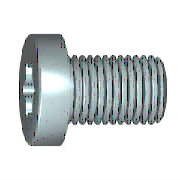
# Autodesk Inventor part: NF E 25-111 - M8x30 classe proprietà 4.8
Saved by Autodesk Inventor 2022 (Build 260153000, 153)
## iProperties
Created: 2021-02-02
Part Number: NF E 25-111 - M8x30 classe proprietà 4.8
Material: Acciaio, Dolce
Description: Testa svasata con impronta a sei lobi - Grado prodotto A - Simbolo CZX
Document SubType Name: Modeling
Standard: NF E 25-111
Designer: Elia
Standards Organization: AFNOR
Language: it-IT
Size Designation: M8x30 classe proprietà 4.8
Categories: <MemberInstance><Categories><Category DisplayName="Elementi di fissaggio" InternalName="e4da775c-781d-43d5-af7c-5136215cf5a6" Mnemonic="FSTN"><Category DisplayName="Bulloni" InternalName="536e6df0-f778-49ac-b2f2-25c71d2aa0b2" Mnemonic="SCRW"><CategoryParameter DisplayName="Designazione diametro nominale" InternalName="03caf894-eafd-4c09-a035-916ac084b87b" Mnemonic="nomdiadesig"/><CategoryParameter DisplayName="Lunghezza nominale" InternalName="238ecbaf-3e6c-45dd-aa95-4068c8e0fd02" Mnemonic="nomlen"/><CategoryParameter DisplayName="Designazione filettatura" InternalName="586d5e89-370a-4089-914f-0110033585c7" Mnemonic="thrdesign"/><CategoryParameter DisplayName="Designazione serie filettatura" InternalName="87c5849c-b3a5-4c3e-9c9b-2feecef9be86" Mnemonic="thrserdsgn"/><CategoryParameter DisplayName="Diametro nominale" InternalName="8bbe3f8e-44cf-40a9-a251-3a6edc8168d6" Mnemonic="nomdia"/><CategoryParameter DisplayName="Tipo filetto" InternalName="b4bbb7bc-d6aa-4c9f-a9a9-4152b9f6fe49" Mnemonic="thrtype"/><CategoryParameter DisplayName="Passo filettatura" InternalName="bb82302e-82d8-4176-8fc1-c5d7bb17d5ad" Mnemonic="pitch1"/><CategoryParameter DisplayName="Filettature per unità" InternalName="bdc6e7d2-ffd0-4d9c-a173-16b95ebb912d" Mnemonic="thrperunit1"/><CategoryParameter DisplayName="Classe filettatura" InternalName="ebc0d23b-2cc6-4d2a-b376-d52aae53bab6" Mnemonic="thrclss"/><Category DisplayName="Testa incassata" InternalName="55e06bf3-7e58-486c-bbdc-745fcc60664d" Mnemonic="CLSCRW"><CategoryParameter DisplayName="Diametro albero" InternalName="179dbae3-102f-48bb-85fe-1e3ecd34f7cc" Mnemonic="grpdia"/><CategoryParameter DisplayName="Lunghezza filettatura" InternalName="3268731d-5f9a-4750-8b01-4a959c46fbf2" Mnemonic="thrlen"/><CategoryParameter DisplayName="Diametro testa" InternalName="46177176-dbdd-4a1b-aefd-4c60c45016af" Mnemonic="headdia"/><CategoryParameter DisplayName="Lunghezza grip" InternalName="52eab69f-422f-4795-9995-175a1b827e67" Mnemonic="grplen"/><CategoryParameter DisplayName="Tipo" InternalName="59a7e495-7a0c-4a5c-bdfd-c090c5f6e2db" Mnemonic="type"/><CategoryParameter DisplayName="Altezza testa" InternalName="99c92c4c-4a02-4ebe-9e64-948fb169e19e" Mnemonic="headh"/></Category></Category></Category><Category DisplayName="TipoDati" InternalName="23b78d0f-2648-40c6-8793-ca6db495c9e8" Mnemonic="DATATYPE"><CategoryParameter DisplayName="NomeVisualizzazione" InternalName="05415f3d-3907-474b-a020-eb9d644f4cf3" Mnemonic="DISPLAYNAME"/><CategoryParameter DisplayName="Norme" InternalName="0c0a119c-1e12-4c84-803f-101930972f5e" Mnemonic="STANDARD"/><CategoryParameter DisplayName="Descrizione" InternalName="13903e3d-64b1-4950-80da-f627842ea37f" Mnemonic="DESCRIPTION"/><CategoryParameter DisplayName="Designazione" InternalName="2675968c-4ce5-49e0-a4f5-552d29089031" Mnemonic="DESIGNATION"/><CategoryParameter DisplayName="Riga di default" InternalName="2af9ec52-faaa-4026-b378-f9fa4afca842" Mnemonic="DEFAULTROW"/><CategoryParameter DisplayName="Nome cartella" InternalName="3f06958e-8713-4116-9be7-ed6184ecc97b" Mnemonic="FOLDERNAME"/><CategoryParameter DisplayName="Guid revisione" InternalName="45a75005-10b1-4dfc-8d6d-dfe629f0b93c" Mnemonic="REVISIONGUID"/><CategoryParameter DisplayName="NomeFile" InternalName="8b46a4cc-9585-4fed-90c3-899f57e09a73" Mnemonic="FILENAME"/><CategoryParameter DisplayName="SocietàNorme" InternalName="8f5914e1-4693-403f-8ab5-d37768198c9d" Mnemonic="STDSORG"/><CategoryParameter DisplayName="Versione famiglia" InternalName="914462f6-6e19-4b14-ba84-155b9680b1d0" Mnemonic="FAMILYREVISION"/><CategoryParameter DisplayName="Revisione norme" InternalName="91d5a463-65c2-4fde-b823-3b7fea5e8e17" Mnemonic="STANDARDREVISION"/><CategoryParameter DisplayName="Revisione membro" InternalName="a65d44b9-392f-4f4f-857b-e4b3d54996fe" Mnemonic="MEMBERREVISION"/><CategoryParameter DisplayName="FormatoPianoRitaglio" InternalName="bc51e27b-3422-4e78-93ef-cec197ddf230" Mnemonic="CLIPFORMAT"/><CategoryParameter DisplayName="Produttore" InternalName="cd6c7a72-a28a-4e50-99a9-2c7f4e13e5ad" Mnemonic="MANUFACTURER"/><CategoryParameter DisplayName="NomeInterno" InternalName="cf1d0246-76d9-4b4a-8305-fa0409afb5c1" Mnemonic="INTERNALNAME"/><CategoryParameter DisplayName="Èmetrico" InternalName="e2385c5b-1ea4-4823-96a8-8de651266ec3" Mnemonic="ISMETRIC"/><Category DisplayName="Parte" InternalName="c0e0b642-3bcb-4cc8-9e80-f96d35c4afa4" Mnemonic="PART"><CategoryParameter DisplayName="Numero parte" InternalName="016b6077-bfbe-49bd-92c9-d8d59c39c941" Mnemonic="PARTNUMBER"/><CategoryParameter DisplayName="Numero di magazzino" InternalName="4dba7c1c-e26c-444e-836c-b08b433409a8" Mnemonic="STOCKNUMBER"/><CategoryParameter DisplayName="Chiave materiale" InternalName="5c9a8adb-dd2b-4535-b97f-0a94a95fe41f" Mnemonic="MATERIALKEY"/><CategoryParameter DisplayName="Materiale" InternalName="818a152a-d3c3-49ca-80ee-df7d91421b8e" Mnemonic="MATERIAL"/></Category></Category><Category DisplayName="MappaPrecedente" InternalName="cd87c42b-3e48-431e-b5c0-1cbeb14dfe77" Mnemonic="LEGACYMAP"><CategoryParameter DisplayName="ID membro DA univoco" InternalName="0918ad47-427f-4fed-ae26-24c81c58f590" Mnemonic="DACOOKIE"/><CategoryParameter DisplayName="Unisci11 ID" InternalName="0ee8fb18-e2ed-4f39-96f6-1f4b5f50aa71" Mnemonic="MERGE11"/><CategoryParameter DisplayName="ID membro CC univoco" InternalName="5193edd4-b2b0-4ab4-9d54-de900eee34e0" Mnemonic="CCCOOKIE"/><CategoryParameter DisplayName="Dividi ID" InternalName="72b5c83c-be7f-45c4-ae51-9160ea6deb26" Mnemonic="SPLIT"/><CategoryParameter DisplayName="IDMembro" InternalName="8e5e0294-fc51-4c8f-b3d7-003dc5ed94f6" Mnemonic="MEMBERID"/><CategoryParameter DisplayName="NomeCatalogo" InternalName="d99d1e27-aa94-4de2-af4c-c348882a6f4f" Mnemonic="CATALOGNAME"/><CategoryParameter DisplayName="NumeroFamiglia" InternalName="e705e1f4-09cb-413e-91f9-551b4188271e" Mnemonic="FAMILYNUMBER"/></Category></Categories><FamilyTemplate Id="si0149"><FamilyTemplateParameters><FamilyTemplateParameter ObjectType="kUserParameterObject" ValueType="xs:double" Id="1" ObjectReferenceKey="GUL"/><FamilyTemplateParameter ObjectType="kUserParameterObject" ValueType="xs:double" Id="2" ObjectReferenceKey="SPD"/><FamilyTemplateParameter ObjectType="kUserParameterObject" ValueType="xs:double" Id="3" ObjectReferenceKey="NLG"/><FamilyTemplateParameter ObjectType="kUserParameterObject" ValueType="xs:double" Id="4" ObjectReferenceKey="KOD"/><FamilyTemplateParameter ObjectType="kUserParameterObject" ValueType="xs:double" Id="5" ObjectReferenceKey="TOA"/><FamilyTemplateParameter ObjectType="kUserParameterObject" ValueType="xs:double" Id="6" ObjectReferenceKey="GD1"/><FamilyTemplateParameter ObjectType="kUserParameterObject" ValueType="xs:double" Id="7" ObjectReferenceKey="GEL"/><FamilyTemplateParameter ObjectType="kUserParameterObject" ValueType="xs:double" Id="8" ObjectReferenceKey="SW"/><FamilyTemplateParameter ObjectType="kUserParameterObject" ValueType="xs:double" Id="9" ObjectReferenceKey="THREADDIA"/><FamilyTemplateParameter ObjectType="kUserParameterObject" ValueType="xs:double" Id="10" ObjectReferenceKey="INTI"/><FamilyTemplateParameter ObjectType="kUserParameterObject" ValueType="xs:double" Id="11" ObjectReferenceKey="BDM"/><FamilyTemplateParameter ObjectType="kUserParameterObject" ValueType="xs:double" Id="12" ObjectReferenceKey="RR"/><FamilyTemplateParameter ObjectType="kUserParameterObject" ValueType="xs:double" Id="13" ObjectReferenceKey="KOH"/><FamilyTemplateParameter ObjectType="kUserParameterObject" ValueType="xs:double" Id="14" ObjectReferenceKey="TPU"/><FamilyTemplateParameter ObjectType="kUserParameterObject" ValueType="xs:double" Id="15" ObjectReferenceKey="PTC"/><FamilyTemplateParameter ObjectType="kUserParameterObject" ValueType="xs:double" Id="16" ObjectReferenceKey="NND"/><FamilyTemplateParameter ObjectType="kUserParameterObject" ValueType="xs:double" Id="17" ObjectReferenceKey="GD"/><FamilyTemplateParameter ObjectType="kUserParameterObject" ValueType="xs:double" Id="18" ObjectReferenceKey="RRK"/><FamilyTemplateParameter ObjectType="kUserParameterObject" ValueType="xs:double" Id="19" ObjectReferenceKey="GAL"/><FamilyTemplateParameter ObjectType="kUserParameterObject" ValueType="xs:double" Id="20" ObjectReferenceKey="E0"/><FamilyTemplateParameter ObjectType="kPropertyObject" ValueType="xs:string" Id="100" ObjectReferenceKey="{32853F0F-3444-11d1-9E93-0060B03C1CA6}" SubObjectId="52"/><FamilyTemplateParameter ObjectType="kPropertyObject" ValueType="xs:string" Id="105" ObjectReferenceKey="{32853F0F-3444-11d1-9E93-0060B03C1CA6}" SubObjectId="5"/><FamilyTemplateParameter ObjectType="kPartComponentDefinitionObject" ValueType="xs:string" Id="110" SubObjectId="Material"/><FamilyTemplateParameter ObjectType="kThreadFeatureObject" ValueType="xs:structure" Id="300" ObjectReferenceKey="1002000010000000a2070000000000008000000000000000" SubObjectId="ThreadInfo"><FamilyTemplateParameter ObjectType="" ValueType="xs:string" Id="301" SubObjectId="ThreadDesignation"/><FamilyTemplateParameter ObjectType="" ValueType="xs:string" Id="302" SubObjectId="ThreadType"/><FamilyTemplateParameter ObjectType="" ValueType="xs:string" Id="303" SubObjectId="ThreadClass"/></FamilyTemplateParameter></FamilyTemplateParameters></FamilyTemplate><CategoryParameterMap><ParamToTemplateMap><ParamToTemplate CategoryParameter="//CategoryParameter[@InternalName='05415f3d-3907-474b-a020-eb9d644f4cf3']" ConstantValue="NF E 25-111"/><ParamToTemplate CategoryParameter="//CategoryParameter[@InternalName='cf1d0246-76d9-4b4a-8305-fa0409afb5c1']" ConstantValue="aaf19020-bd3f-477f-9127-f56056b857a9"/><ParamToTemplate CategoryParameter="//CategoryParameter[@InternalName='3f06958e-8713-4116-9be7-ed6184ecc97b']" ConstantValue="NF E 25-111"/><ParamToTemplate CategoryParameter="//CategoryParameter[@InternalName='914462f6-6e19-4b14-ba84-155b9680b1d0']" ConstantValue="10"/><ParamToTemplate CategoryParameter="//CategoryParameter[@InternalName='bc51e27b-3422-4e78-93ef-cec197ddf230']" ConstantValue="CF_INVENTOR.STDPARTS"/><ParamToTemplate CategoryParameter="//CategoryParameter[@InternalName='e2385c5b-1ea4-4823-96a8-8de651266ec3']" ConstantValue="true"/><ParamToTemplate CategoryParameter="//CategoryParameter[@InternalName='13903e3d-64b1-4950-80da-f627842ea37f']" ConstantValue="Six lobes recessed countersunk head - Product grade A - Symbol CZX"/><ParamToTemplate CategoryParameter="//CategoryParameter[@InternalName='8f5914e1-4693-403f-8ab5-d37768198c9d']" ConstantValue="AFNOR"/><ParamToTemplate CategoryParameter="//CategoryParameter[@InternalName='0c0a119c-1e12-4c84-803f-101930972f5e']" ConstantValue="NF E 25-111"/><ParamToTemplate CategoryParameter="//CategoryParameter[@InternalName='cd6c7a72-a28a-4e50-99a9-2c7f4e13e5ad']" TemplateParameter="104"/><ParamToTemplate CategoryParameter="//CategoryParameter[@InternalName='91d5a463-65c2-4fde-b823-3b7fea5e8e17']" TemplateParameter="103"/><ParamToTemplate CategoryParameter="//CategoryParameter[@InternalName='45a75005-10b1-4dfc-8d6d-dfe629f0b93c']" ConstantValue="6c897606-b0fe-47f7-a520-b4065de4669e"/><ParamToTemplate CategoryParameter="//CategoryParameter[@InternalName='2af9ec52-faaa-4026-b378-f9fa4afca842']" ConstantValue="10"/><ParamToTemplate CategoryParameter="//CategoryParameter[@InternalName='d99d1e27-aa94-4de2-af4c-c348882a6f4f']" ConstantValue="AFNOR"/><ParamToTemplate CategoryParameter="//CategoryParameter[@InternalName='e705e1f4-09cb-413e-91f9-551b4188271e']" ConstantValue="18"/><ParamToTemplate CategoryParameter="//CategoryParameter[@InternalName='8b46a4cc-9585-4fed-90c3-899f57e09a73']" ConstantValue="NF E 25-111 - M8x30 classe proprietà 4.8"/><ParamToTemplate CategoryParameter="//CategoryParameter[@InternalName='a65d44b9-392f-4f4f-857b-e4b3d54996fe']" ConstantValue="72F727D1-4201-4A58-904D-8504DE5D0C6A"/><ParamToTemplate CategoryParameter="//CategoryParameter[@InternalName='52eab69f-422f-4795-9995-175a1b827e67']" ConstantValue="1,25"/><ParamToTemplate CategoryParameter="//CategoryParameter[@InternalName='ebc0d23b-2cc6-4d2a-b376-d52aae53bab6']" ConstantValue="6g"/><ParamToTemplate CategoryParameter="//CategoryParameter[@InternalName='03caf894-eafd-4c09-a035-916ac084b87b']" ConstantValue="M8"/><ParamToTemplate CategoryParameter="//CategoryParameter[@InternalName='b4bbb7bc-d6aa-4c9f-a9a9-4152b9f6fe49']" ConstantValue="ISO Metric profile"/><ParamToTemplate CategoryParameter="//CategoryParameter[@InternalName='8e5e0294-fc51-4c8f-b3d7-003dc5ed94f6']" ConstantValue="690"/><ParamToTemplate CategoryParameter="//CategoryParameter[@InternalName='179dbae3-102f-48bb-85fe-1e3ecd34f7cc']" TemplateParameter="11"/><ParamToTemplate CategoryParameter="//CategoryParameter[@InternalName='2675968c-4ce5-49e0-a4f5-552d29089031']" TemplateParameter="100"/><ParamToTemplate CategoryParameter="//CategoryParameter[@InternalName='3268731d-5f9a-4750-8b01-4a959c46fbf2']" TemplateParameter="7"/><ParamToTemplate CategoryParameter="//CategoryParameter[@InternalName='46177176-dbdd-4a1b-aefd-4c60c45016af']" TemplateParameter="4"/><ParamToTemplate CategoryParameter="//CategoryParameter[@InternalName='99c92c4c-4a02-4ebe-9e64-948fb169e19e']" TemplateParameter="13"/><ParamToTemplate CategoryParameter="//CategoryParameter[@InternalName='818a152a-d3c3-49ca-80ee-df7d91421b8e']" TemplateParameter="110"/><ParamToTemplate CategoryParameter="//CategoryParameter[@InternalName='238ecbaf-3e6c-45dd-aa95-4068c8e0fd02']" TemplateParameter="3"/><ParamToTemplate CategoryParameter="//CategoryParameter[@InternalName='8bbe3f8e-44cf-40a9-a251-3a6edc8168d6']" TemplateParameter="16"/><ParamToTemplate CategoryParameter="//CategoryParameter[@InternalName='016b6077-bfbe-49bd-92c9-d8d59c39c941']" TemplateParameter="105"/><ParamToTemplate CategoryParameter="//CategoryParameter[@InternalName='bb82302e-82d8-4176-8fc1-c5d7bb17d5ad']" TemplateParameter="15"/><ParamToTemplate CategoryParameter="//CategoryParameter[@InternalName='586d5e89-370a-4089-914f-0110033585c7']" TemplateParameter="301"/><ParamToTemplate CategoryParameter="//CategoryParameter[@InternalName='bdc6e7d2-ffd0-4d9c-a173-16b95ebb912d']" TemplateParameter="14"/></ParamToTemplateMap></CategoryParameterMap></MemberInstance>
Density: 7.85 g/cm^3
Appearance: Semilucidato
IsCustomPart: 0
Author: Elia
Autodesk Inventor part; units mm, degrees
ref_plane "YZ Plane" through (0, 0, 0) normal (1, 0, 0) x (0, 1, 0)
ref_plane "XZ Plane" through (0, 0, 0) normal (0, 1, 0) x (-1, 0, 0)
sketch "Schizzo1" plane through (0, 0, 0) normal (0, 0, 1) x (1, 0, 0)
  line L0 (0.345, 0) -> (30, 0)
  line L1 (30, 0) -> (30, 4)
  line L2 (30, 4) -> (1.25, 4)
  line L3 (1.25, 4) -> (0.4832, 3.6615)
  line L4 (0.4832, 3.6615) -> (0, 3.6615)
  line L5 (0, 3.6615) -> (0, 6.5)
  line L6 (0, 6.5) -> (-5, 6.5)
  line L7 (-5, 6.5) -> (-5, 3.975)
  line L8 (-5, 3.975) -> (-1.95, 3.975)
  line L9 (-1.95, 3.975) -> (0.345, 0)
  line L10 (-12, 0) -> (37, 0) projected
  line L11 (0, -1.3) -> (0, 7.8) projected
  line L12 (1.25, 4) -> (0, 4) construction
  dimension "d1" = 28.75
  dimension "d2" = 0.7668
  dimension "d3" = 5
  dimension "d4" = 3.05
  dimension "d5" = 60
  dimension "d6" = 8
  dimension "d7" = 7.323
  dimension "d8" = 7.95
  dimension "d9" = 13
  dimension "d20" = 30
  constraints: 22 end point, 6 parallel, 2 collinear, 2 perpendicular, 1 horizontal, 1 point on line
  measures "d1" distance from line of L2.end L1
  measures "d2" horizontal distance of L3.end L2.end
  measures "d3" distance between parallel lines of L7 L5
  measures "d4" distance of L7.end L8.end
  measures "d5" angle of L9 L0
  measures "d6" diameter of L2 L0
  measures "d7" diameter of L4 L0
  measures "d8" diameter of L8 L0
  measures "d9" diameter of L6 L0
  measures "d20" distance between parallel lines of L1 L5
revolve "Corpo" add sketch "Schizzo1" angle 360 about axis through (0.345, 0, 0) along (1, 0, 0) contours L9 L11 L4 L3 L2 L1 L0 | L9 L8 L7 L6 L5 L11
sketch "Schizzo2" plane through (-5, 0, 0) normal (-1, 0, 0) x (0, 0, 1)
  line L0 (0, -9.1) -> (0, 9.1) projected
  line L1 (-9.1, 0) -> (9.1, 0) projected
  circle A0 centre (0, 0) radius 3.975 construction
  circle A1 centre (0, 0) radius 2.82 construction
  line L2 (0, 0) -> (3.4425, 1.9875) construction
  line L3 (0, 0) -> (1.9875, 3.4425) construction
  arc A2 (2.2571, 2.795) -> (1.292, 3.3522) centre (1.6988, 2.9423) ccw
  arc A3 (2.2571, 2.795) -> (3.5491, 0.5572) centre (4.0306, 2.3271) ccw
  arc A4 (3.5491, -0.5572) -> (3.5491, 0.5572) centre (3.3975, 0) ccw
  arc A5 (3.5491, -0.5572) -> (2.2571, -2.795) centre (4.0306, -2.3271) ccw
  arc A6 (-1.292, 3.3522) -> (1.292, 3.3522) centre (0, 4.6542) ccw
  arc A7 (-1.292, 3.3522) -> (-2.2571, 2.795) centre (-1.6988, 2.9423) ccw
  arc A8 (-3.5491, 0.5572) -> (-2.2571, 2.795) centre (-4.0306, 2.3271) ccw
  arc A9 (-3.5491, 0.5572) -> (-3.5491, -0.5572) centre (-3.3975, 0) ccw
  arc A10 (-2.2571, -2.795) -> (-3.5491, -0.5572) centre (-4.0306, -2.3271) ccw
  arc A11 (1.292, -3.3522) -> (2.2571, -2.795) centre (1.6988, -2.9423) ccw
  arc A12 (1.292, -3.3522) -> (-1.292, -3.3522) centre (0, -4.6542) ccw
  arc A13 (-2.2571, -2.795) -> (-1.292, -3.3522) centre (-1.6988, -2.9423) ccw
  circle A14 centre (0, 0) radius 3.975 projected
  dimension "d34" = 30
  dimension "d35" = 60
  dimension "d36" = 5.64
  dimension "d37" = 7.95
  dimension "d38" = 0.5775
  constraints: 26 point on circle, 17 symmetric about line, 14 centre point, 7 tangent, 4 end point, 4 point on line, 2 coincident, 8 other
  measures "d34" angle of L1 L2
  measures "d35" angle of L1 L3
  measures "d36" diameter of A1
  measures "d37" diameter of A0
  measures "d38" radius of A2
extrude "Intaglio" add sketch "Schizzo2" against normal blind 3.05 contours A14 A13 A12 L0 | L0 A12 A11 A14 | A14 A9 A10 A13 | A11 A5 A4 A14 | A14 A7 A8 A9 | A4 A3 A2 A14 | A6 A7 A14 L0 | L0 A14 A2 A6
fillet "Raccordo1" radius 0.4 1 edges at (-5, -6.5, 0)
thread "Filettatura" size "M8x1.25" class "6g" standard "ISO Metric profile" length 28.75
chamfer "Smusso1" distance 0.4704 distance2 0.7669 1 edges at (30, -4, 0) measured on face at (30, -0.4013, -0.6579)
ref_plane "Work Plane1" through (15.625, 0, 0) normal (0, -0.6399, -0.7684) x (1, 0, 0)
equation "\"d1\" = GEL"
equation "\"d2\" = GAL"
equation "\"d3\" = KOH"
equation "\"d4\" = INTI"
equation "\"d6\" = GD"
equation "\"d7\" = BDM"
equation "\"d8\" = SW"
equation "\"d9\" = KOD"
equation "\"d20\" = NLG"
equation "\"d36\" = E0"
equation "\"d37\" = SW"
equation "\"d38\" = -0.25 * E0 + 0.25 * SW"
equation "\"d11\" = INTI"
equation "\"d17\" = RR"
equation "\"d13\" = GEL"
equation "\"d15\" = -0.5 * SPD + 0.5 * GD"
equation "\"GD\" = NND"
equation "\"NLG\" = 30"
equation "\"GEL\" = 28.75"
equation "\"KOD\" = 13"
equation "\"KOH\" = 5"
equation "\"INTI\" = 3.05"
equation "\"GAL\" = 0.61345 * PTC"
equation "\"GUL\" = 0.61345 * PTC"
equation "\"BDM\" = 7.323"
equation "\"SW\" = 7.95"
equation "\"RR\" = 0.4"
equation "\"SPD\" = NND - 1.2269 * GAL"
equation "\"E0\" = 5.64"
equation "\"TOA\" = 30deg"
equation "\"GD1\" = THREADDIA - 1.2269 * PTC"
equation "\"THREADDIA\" = 8"
equation "\"PTC\" = 1.25"
equation "\"NND\" = 8"
equation "\"RRK\" = 0.548"
body "Solid1"
